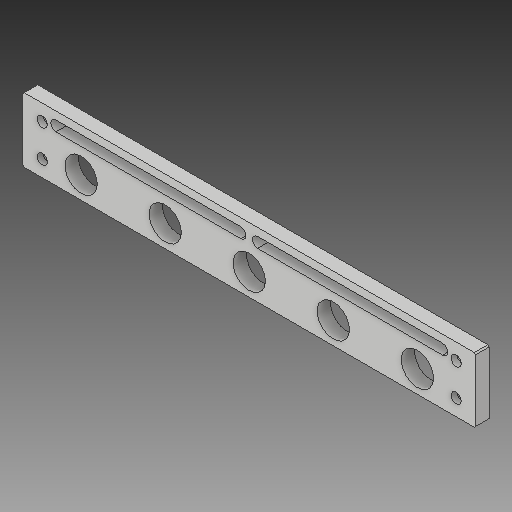
# Autodesk Inventor part: SuportePincasBlocoFabricado
Saved by Autodesk Inventor 2018 (Build 220112000, 112)
## iProperties
Created: 2018-08-27
Part Number: SuportePincasBlocoFabricado
Material: Genérico
Document SubType Name: Modeling
Designer: Georgines
Density: 1 g/cm^3
Appearance: Padrão
Mass: 131.672 g
Surface Area: 449.962 cm^2
Volume: 131.672 cm^3
Author: Georgines
Autodesk Inventor part; units mm, degrees
ref_plane "YZ Plane" through (0, 0, 0) normal (1, 0, 0) x (0, 1, 0)
ref_plane "XZ Plane" through (0, 0, 0) normal (0, 1, 0) x (-1, 0, 0)
ref_plane "XY Plane" through (0, 0, 0) normal (0, 0, 1) x (1, 0, 0)
sketch "Esboço1" plane through (0, 0, 0) normal (0, 0, 1) x (1, 0, 0)
  line L0 (-293, 0) -> (-323, 0) construction
  line L1 (-323, 0) -> (-323, 50) construction
  line L2 (27, 0) -> (27, 50) construction
  line L3 (27, 0) -> (0, 0) construction
  line L4 (-3, 50) -> (27, 50) construction
  line L5 (-323, 50) -> (-293, 50) construction
  line L6 (27, 0) -> (-323, 0)
  line L7 (-323, 0) -> (-323, 50)
  line L8 (-323, 50) -> (27, 50)
  line L9 (27, 50) -> (27, 0)
  constraints: 8 end point, 2 parallel, 1 horizontal, 1 perpendicular
extrude "bloco principal" add sketch "Esboço1" along normal blind 10.5
sketch "Esboço4" plane through (0, 0, 10.5) normal (0, 0, 1) x (1, 0, 0)
  line L0 (27, 0) -> (27, 50) projected
  line L1 (27, 40) -> (-323, 40) construction
  line L2 (-323, 50) -> (-323, 0) projected
  line L3 (5.5, 40) -> (-145.5, 40) construction
  line L4 (1.5, 44) -> (-141.5, 44)
  line L5 (-141.5, 36) -> (1.5, 36)
  arc A0 (1.5, 36) -> (1.5, 44) centre (1.5, 40) ccw
  arc A1 (-141.5, 44) -> (-141.5, 36) centre (-141.5, 40) ccw
  line L6 (-150.5, 40) -> (-301.5, 40) construction
  line L7 (-154.5, 44) -> (-297.5, 44)
  line L8 (-297.5, 36) -> (-154.5, 36)
  arc A2 (-154.5, 36) -> (-154.5, 44) centre (-154.5, 40) ccw
  arc A3 (-297.5, 44) -> (-297.5, 36) centre (-297.5, 40) ccw
  line L9 (-323, 0) -> (27, 0) projected
  line L10 (27, 50) -> (-323, 50) projected
  point P0 (0, 0)
  point P1 (-70, 40)
  point P2 (-226, 40)
  dimension "d39" = 97
  dimension "d40" = 97
  dimension "d41" = 8
  dimension "d42" = 8
  dimension "d43" = 143
  dimension "d44" = 143
  dimension "d46" = 10
  constraints: 18 end point, 12 point on circle, 10 point on line, 8 tangent, 4 centre point, 2 midpoint, 2 parallel, 1 horizontal
  measures "d39" distance from line of point (-226, 40) L2
  measures "d40" distance from line of L0 point (-70, 40)
  measures "d41" distance between parallel lines of L4 L5
  measures "d42" distance between parallel lines of L7 L8
  measures "d43" distance of A2.centre A3.centre
  measures "d44" distance of A0.centre A1.centre
  measures "d46" distance between parallel lines of L10 L1
extrude "fenda" cut sketch "Esboço4" against normal through all contours A0 L5 A1 L4 | A2 L8 A3 L7
sketch "Esboço5" plane through (0, 0, 10.5) normal (0, 0, 1) x (1, 0, 0)
  line L0 (27, 0) -> (27, 50) projected
  line L1 (27, 17) -> (-323, 17) construction
  line L2 (-323, 50) -> (-323, 0) projected
  circle A0 centre (-148, 17) radius 12.5
  circle A1 centre (-213, 17) radius 12.5
  circle A2 centre (-278, 17) radius 12.5
  circle A3 centre (-83, 17) radius 12.5
  circle A4 centre (-148, 17) radius 12.5 construction
  circle A5 centre (-213, 17) radius 12.5 construction
  circle A6 centre (-18, 17) radius 12.5
  circle A7 centre (-83, 17) radius 12.5 construction
  circle A8 centre (-148, 17) radius 12.5 construction
  line L3 (-323, 0) -> (27, 0) projected
  point P0 (0, 0)
  dimension "d51" = 65
  dimension "d54" = 65
  dimension "d57" = 17
  dimension "d58" = 25
  constraints: 9 centre point, 3 horizontal, 2 end point, 2 point on line, 1 midpoint, 16 other
  measures "d51" distance of A0.centre A1.centre
  measures "d54" distance of A0.centre A3.centre
  measures "d57" distance between parallel lines of L3 L1
  measures "d58" diameter of A0
extrude "furos traseiros" cut sketch "Esboço5" against normal through all
sketch "Esboço6" plane through (0, 0, 10.5) normal (0, 0, 1) x (1, 0, 0)
  circle A0 centre (-308, 12.5) radius 1.621 construction
  circle A1 centre (-308, 37.5) radius 1.621 construction
  circle A2 centre (12, 12.5) radius 1.621 construction
  circle A3 centre (12, 37.5) radius 1.621 construction
  point P0 (0, 0)
hole "furos fixação" at (-308, 12.5, 10.5) at (-308, 37.5, 10.5) at (12, 12.5, 10.5) at (12, 37.5, 10.5) direction (0, 0, -1) diameter 4 end through all counterbore diameter 8 counterbore depth 4.5
chamfer "Chanfro1" distance 1 angle 45 4 edges at (27, 0, 5.25) (27, 50, 5.25) (-323, 50, 5.25) (-323, 0, 5.25)
equation "\"d40\" = d39"
equation "\"d41\" = d42"
equation "\"d44\" = d43"
